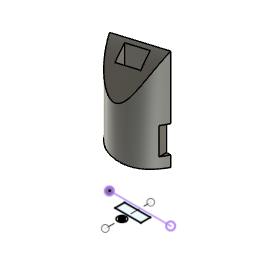
Back Hand Exo Top v2 v5 (Autodesk Fusion 360 design; units mm, degrees)
Autodesk Fusion 360 part; units mm, degrees
ref_plane "WorkPlane3" through (54.5653, 17.8993, 37.432) normal (0, 1, 0) x (-1, 0, 0)
sketch "Top part base" plane through (54.5653, 17.8993, 37.432) normal (0, 1, 0) x (1, 0, 0)
  line L0 (22.5, -74.3) -> (22.5, 0)
  line L1 (22.5, 0) -> (-22.5, -5.2067)
  line L2 (-22.5, -5.2067) -> (-22.5, -63.7067)
  line L3 (-22.5, -63.7067) -> (22.5, -74.3)
  line L4 (-30, 0) -> (100, 0) construction
  line L5 (0, -120.4179) -> (0, 0) construction
  dimension "d112" = 45
  dimension "d113" = 58.5
  dimension "d114" = 74.3
  dimension "d115" = 6.6
  dimension "d136" = 22.5
  constraint vertical L0
  constraint parallel L0 L2
  constraint horizontal L4
  constraint vertical L5
  constraint coincident L5.end origin
  constraint coincident L5.end L4
  constraint coincident L0.end L4
  measures "d112" distance of L0 L2
  measures "d113" distance of L1.end L2.end
  measures "d114" distance of L0.start L0.end
  measures "d115" angle of L1 L4
  measures "d136" distance of L0 L5
extrude "Extrude9" add sketch "Top part base" along normal blind 26
sketch "Strap holes" plane through (0, 17.8993, 0) normal (0, -1, 0) x (1, 0, 0)
  line L0 (32.0653, 101.1387) -> (32.0653, 42.6387)
  line L1 (32.0653, 42.6387) -> (77.0653, 37.432)
  line L2 (77.0653, 37.432) -> (77.0653, 111.732)
  line L3 (77.0653, 111.732) -> (32.0653, 101.1387)
  line L4 (32.0653, 65.432) -> (35.0653, 65.432)
  line L5 (35.0653, 65.432) -> (35.0653, 45.432)
  line L6 (35.0653, 45.432) -> (32.0653, 45.432)
  line L7 (32.0653, 45.432) -> (32.0653, 65.432)
  line L8 (74.0653, 65.432) -> (77.0653, 65.432)
  line L9 (77.0653, 65.432) -> (77.0653, 45.432)
  line L10 (77.0653, 45.432) -> (74.0653, 45.432)
  line L11 (74.0653, 45.432) -> (74.0653, 65.432)
  dimension "d127" = 20
  dimension "d128" = 8
  dimension "d129" = 3
  constraint horizontal L4
  constraint vertical L5
  constraint horizontal L6
  constraint vertical L7
  constraint horizontal L8
  constraint vertical L9
  constraint horizontal L10
  constraint vertical L11
  constraint equal L5 L9
  constraint collinear L6 L10
  constraint equal L6 L10
  constraint collinear L2 L9
  constraint collinear L0 L7
  measures "d127" distance of L8.end L9.end
  measures "d128" vertical distance of L1.end L6.end
  measures "d129" distance of L9.end L10.end
ref_plane "WorkPlane4" through (77.0653, 30.8993, 74.582) normal (1, 0, 0) x (0, 0, -1)
sketch "Sagittal cut" plane through (77.0653, 32.8993, 74.582) normal (1, 0, 0) x (0, 1, 0)
  spline S0 degree 5 poles (-15, -37.15) (-14.8228, -35.1184) (-14.4401, -31.1002) (-13.7813, -25.2077) (-12.7308, -17.6251) (-11.1096, -8.6371) (-9.1479, -0.1911) (-6.8088, 7.6542) (-4.0594, 14.8463) (-0.8903, 21.3705) (2.6783, 27.2588) (5.8319, 31.4939) (8.3554, 34.4183) (10.1069, 36.2578) (11, 37.15) knots 0 0 0 0 0 0 0.1 0.2 0.3 0.4 0.5 0.6 0.7 0.8 0.9 1 1 1 1 1 1
  line L0 (11, 37.15) -> (11, 47.8614)
  line L1 (11, 47.8614) -> (-36.1325, 47.8614)
  line L2 (-36.1325, 47.8614) -> (-36.1325, -43.6471)
  line L3 (-36.1325, -43.6471) -> (-15, -37.15)
  line L4 (11, 37.15) -> (11, -37.15)
  line L5 (-15, 37.15) -> (11, 37.15)
  point P0 (-5, 12.15)
  point P1 (11, 37.15)
  point P2 (-15, -37.15)
  dimension "d138" = 16
  dimension "d139" = 25
  constraint vertical L0
  constraint perpendicular L0 L1
  constraint perpendicular L1 L2
  constraint coincident P1 S0.end
  constraint coincident P2 S0.start
  measures "d138" distance of P0 L4
  measures "d139" distance of P0 L5
sketch "Coronal cut" plane through (0, 0, 0) normal (0, 0, 1) x (1, 0, 0)
  spline S0 degree 5 poles (31.7376, 44.322) (32.5022, 42.5207) (34.0775, 39.1802) (36.5786, 34.9567) (40.168, 30.8144) (44.9604, 27.6886) (49.9104, 26.1323) (54.8705, 25.7484) (59.7217, 26.3447) (64.4037, 28.0555) (68.8948, 31.2302) (72.3351, 35.2946) (74.8332, 39.3813) (76.4629, 42.5938) (77.2689, 44.322) knots 0 0 0 0 0 0 0.1 0.2 0.3 0.4 0.5 0.6 0.7 0.8 0.9 1 1 1 1 1 1
  line L0 (74.0992, 37.5247) -> (80.4385, 51.1193)
  line L1 (28.8071, 51.2258) -> (34.668, 37.4183)
  line L2 (31.7376, 44.322) -> (23, 44.322)
  line L3 (23, 44.322) -> (23, 6)
  line L4 (23, 6) -> (82, 6)
  line L5 (82, 6) -> (82, 44.322)
  line L6 (82, 44.322) -> (77.2689, 44.322)
  line L7 (98, 50) -> (26, 50) construction
  point P0 (55, 26)
  dimension "d161" = 15
  dimension "d162" = 15
  dimension "d163" = 67
  dimension "d164" = 65
  constraint midpoint S0.end L0
  constraint midpoint S0.start L1
  constraint horizontal L2
  constraint perpendicular L2 L3
  constraint perpendicular L3 L4
  constraint perpendicular L4 L5
  constraint perpendicular L5 L6
  constraint collinear L2 L6
  constraint perpendicular L5 L7
  measures "d161" distance of L0.start L0.end
  measures "d162" distance of L1.start L1.end
  measures "d163" angle of L1 L7
  measures "d164" angle of L0 L7
extrude "Extrude14" cut sketch "Coronal cut" along normal blind 125
sweep "Sweep1" cut profiles "Sagittal cut" along 1 edges at (54.5653, 43.8993, 106.4354) section 1
sketch "puck squeezer hole" plane through (0, 0, 0) normal (0, 0, 1) x (1, 0, 0)
  circle A0 centre (54.5653, 30.3993) radius 3
  line L0 (77.0653, 43.8993) -> (32.0653, 43.8993)
  line L1 (32.0653, 43.5634) -> (32.0653, 43.8993)
  line L2 (45.0653, 34.8993) -> (64.0653, 34.8993)
  line L3 (64.0653, 34.8993) -> (64.0653, 41.8993)
  line L4 (64.0653, 41.8993) -> (45.0653, 41.8993)
  line L5 (45.0653, 41.8993) -> (45.0653, 34.8993)
  line L6 (54.5653, 18.1073) -> (54.5653, 51.6914) construction
  dimension "d148" = 13.5
  dimension "d149" = 6
  dimension "d150" = 22.5
  dimension "d154" = 2
  dimension "d155" = 7
  dimension "d156" = 19
  constraint horizontal L2
  constraint vertical L3
  constraint horizontal L4
  constraint vertical L5
  constraint vertical L6
  constraint coincident A0.centre L6
  constraint midpoint L2 L6
  measures "d148" distance of A0.centre L0
  measures "d149" diameter of A0
  measures "d150" distance of A0.centre L1
  measures "d154" distance of L0 L4
  measures "d155" distance of L2.start L4.end
  measures "d156" distance of L2.start L2.end
hole "Hole4" at (54.5653, 30.3993, 0) direction (0, 0, 1) diameter 6 depth 70 tip angle 118
extrude "Extrude15" cut sketch "puck squeezer hole" along normal blind 140 contours L2 L3 L4 L5
extrude "Extrude16" cut sketch "Strap holes" against normal blind 75 contours L0 L4 L5 L6 L7 | L2 L8 L9 L10 L11
equation "d136 = d112 / 2"
